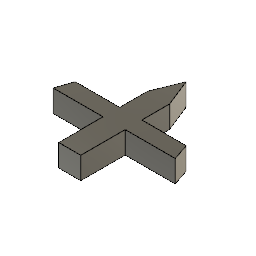
test2 v1 (Autodesk Fusion 360 design; units mm, degrees)
Autodesk Fusion 360 part; units mm, degrees
sketch "Sketch1" plane through (0, 0, 0) normal (0, 0, 1) x (1, 0, 0)
  line L0 (0, 50) -> (-10, 25)
  line L1 (-10, 25) -> (-10, 0)
  line L2 (-50, 0) -> (-10, 0)
  line L3 (0, 50) -> (10, 25)
  line L4 (10, 0) -> (10, 25)
  line L5 (50, 0) -> (10, 0)
  line L6 (-55, -15) -> (-50, 0)
  line L7 (55, -15) -> (50, 0)
  line L8 (-10, -15) -> (-10, -55)
  line L9 (10, -55) -> (10, -15)
  line L10 (-55, -15) -> (-10, -15)
  line L11 (10, -15) -> (55, -15)
  line L12 (-10, -55) -> (10, -55)
  constraint vertical L1
  constraint perpendicular L1 L2
  constraint vertical L4
  constraint perpendicular L4 L5
  constraint parallel L5 L10
  constraint perpendicular L8 L10
  constraint coincident L9.end L10
  constraint perpendicular L9 L10
  constraint collinear L10 L11
  constraint perpendicular L9 L12
extrude "Extrude1" add sketch "Sketch1" along normal blind 20
